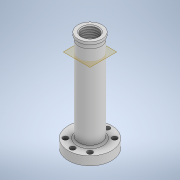
# Autodesk Inventor part: herramienta2
Saved by Autodesk Inventor 2022.2 (Build 262287000, 287)
## iProperties
Created: 2022-06-15
Part Number: herramienta2
Material: Genérico
Document SubType Name: Modeling
Designer: javic
Density: 1 g/cm^3
Appearance: Valor por defecto
Author: javic
Autodesk Inventor part; units mm, degrees
ref_plane "YZ Plane" through (0, 0, 0) normal (1, 0, 0) x (0, 1, 0)
ref_plane "XZ Plane" through (0, 0, 0) normal (0, 1, 0) x (-1, 0, 0)
ref_plane "XY Plane" through (0, 0, 0) normal (0, 0, 1) x (1, 0, 0)
sketch "Boceto1" plane through (0, 0, 0) normal (0, 1, 0) x (-1, 0, 0)
  circle A0 centre (0, 0) radius 25
  circle A1 centre (0, -20) radius 3
  circle A2 centre (-14.1421, -14.1421) radius 3
  circle A3 centre (14.1421, -14.1421) radius 3
  circle A4 centre (0, 20) radius 3
  circle A5 centre (-14.1421, 14.1421) radius 3
  circle A6 centre (14.1421, 14.1421) radius 3
  line L0 (0, -23) -> (0, -28.5119)
  dimension "d2" = 6
  dimension "d0" = 50
  dimension "d4" = 6
  dimension "d6" = 6
  constraints: 6 centre point, 2 end point, 1 coincident, 1 vertical, 1 vertical alignment, 2 other
  measures "d0" diameter of A0
  measures "d4" diameter of A2
  measures "d6" diameter of A3
extrude "Extrusión1" add sketch "Boceto1" along normal blind 10
sketch "Boceto2" plane through (0, 10, 0) normal (0, 1, 0) x (1, 0, 0)
  circle A0 centre (0, 0) radius 9.15
  circle A1 centre (0, 0) radius 13
  dimension "d9" = 18.3
  dimension "d10" = 26
  constraints: 2 centre point, 2 coincident
  measures "d9" diameter of A0
  measures "d10" diameter of A1
extrude "Extrusión2" add sketch "Boceto2" along normal blind 106
fillet "Empalme1" radius 2 1 edges at (-13, 10, 0)
chamfer "Chaflán1" distance 1 angle 45 1 edges at (-9.15, 116, 0)
sketch "Boceto4" plane through (0, 116, 0) normal (0, 1, 0) x (1, 0, 0)
  circle A0 centre (0, 0) radius 11
  circle A1 centre (0, 0) radius 14
  dimension "d22" = 28
  constraints: 2 centre point, 2 coincident
  measures "d22" diameter of A1
extrude "Extrusión4" add sketch "Boceto4" against normal blind 3
fillet "Empalme3" radius 12 1 edges at (-13, 113, 0)
thread "Thread1" size "M6x1" class "6H" standard "ANSI Metric M Profile" full length
thread "Thread2" size "M6x1" class "6H" standard "ANSI Metric M Profile" full length
thread "Thread3" size "M6x1" class "6H" standard "ANSI Metric M Profile" full length
thread "Thread4" size "M6x1" class "6H" standard "ANSI Metric M Profile" full length
thread "Thread5" size "M6x1" class "6H" standard "ANSI Metric M Profile" full length
thread "Thread6" size "M6x1" class "6H" standard "ANSI Metric M Profile" full length
chamfer "Chamfer2" [suppressed]
ref_plane "Work Plane1" through (0, 96, 0) normal (0, 1, 0) x (1, 0, 0)
sketch "Sketch5" plane through (0, 96, 0) normal (0, 1, 0) x (1, 0, 0)
  circle A0 centre (0, 0) radius 13 projected
  circle A1 centre (0, 0) radius 13 projected
  circle A2 centre (0, 0) radius 9.15 projected
  circle A3 centre (0, 0) radius 9.15 projected
  circle A4 centre (0, 0) radius 9.15 projected
  circle A5 centre (0, 0) radius 9.15 projected
  circle A6 centre (0, 0) radius 10.85
  dimension "d43" = 1.7
  constraints: 1 centre point
  measures "d43" radial gap between concentric circles of A2 A6
extrude "Extrusion5" cut sketch "Sketch5" along normal blind 1 contours A6
thread "Thread7" size "M20x2.5" class "6H" standard "ANSI Metric M Profile" full length
